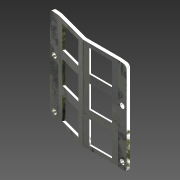
# Autodesk Inventor part: keyplate2
Saved by Autodesk Inventor 2018 (Build 220112000, 112)
## iProperties
Created: 2018-05-25
Part Number: keyplate2
Material: アルミニウム 6061
Document SubType Name: Sheet Metal
Designer: NaMACHAN
Mass: 8.70431 g
Surface Area: 50.6323 cm^2
Volume: 3.22382 cm^3
Density: 2.7 g/cm^3
Flat Pattern Width: 5.7 cm
Flat Pattern Length: 5.44568 cm
Flat Pattern Area: 31.0404 cm^2
Sheet Metal Rule: Al2mm
Sheet Metal Width: 57.000 mm
Sheet Metal Length: 54.457 mm
Sheet Metal Area: 3104.035 mm^2
Appearance: アルミニウム - フラット
Author: NaMACHAN
Autodesk Inventor part; units mm, degrees
ref_plane "YZ Plane" through (0, 0, 0) normal (1, 0, 0) x (0, 1, 0)
ref_plane "XZ Plane" through (0, 0, 0) normal (0, 1, 0) x (-1, 0, 0)
ref_plane "XY Plane" through (0, 0, 0) normal (0, 0, 1) x (1, 0, 0)
sketch "スケッチ1" plane through (0, 0, 0) normal (0, 1, 0) x (-1, 0, 0)
  line L0 (-10.5, -28.5) -> (10.5, -28.5)
  line L1 (10.5, -28.5) -> (10.5, 28.5)
  line L2 (10.5, 28.5) -> (-10.5, 28.5)
  line L3 (-10.5, 28.5) -> (-10.5, -28.5)
  line L4 (-10.5, -28.5) -> (10.5, 28.5) construction
  line L5 (10.5, -28.5) -> (-10.5, 28.5) construction
  line L6 (-7, 12) -> (7, 12)
  line L7 (7, 12) -> (7, 26)
  line L8 (7, 26) -> (-7, 26)
  line L9 (-7, 26) -> (-7, 12)
  line L10 (-7, 12) -> (7, 26) construction
  line L11 (7, 12) -> (-7, 26) construction
  line L12 (-7, -7) -> (7, -7)
  line L13 (7, -7) -> (7, 7)
  line L14 (7, 7) -> (-7, 7)
  line L15 (-7, 7) -> (-7, -7)
  line L16 (-7, -7) -> (7, 7) construction
  line L17 (7, -7) -> (-7, 7) construction
  line L18 (7, -26) -> (-7, -26)
  line L19 (-7, -26) -> (-7, -12)
  line L20 (-7, -12) -> (7, -12)
  line L21 (7, -12) -> (7, -26)
  line L22 (7, -26) -> (-7, -12) construction
  line L23 (-7, -26) -> (7, -12) construction
  point P0 (0, 0)
  point P1 (0, 19)
  point P2 (0, 0)
  point P3 (0, 0)
  point P4 (0, 0)
  point P5 (0, 19)
  point P6 (0, -19)
  point P7 (0, -19)
  dimension "d0" = 21
  dimension "d1" = 57
  dimension "d2" = 14
  dimension "d3" = 14
  dimension "d345" = 14
  dimension "d346" = 14
  dimension "d391" = 19
  dimension "d393" = 19
  dimension "d410" = 14
  dimension "d411" = 14
  dimension "d412" = 19
  measures "d0" distance of L2.end L1.end
  measures "d1" distance of L1.end L0.end
  measures "d2" distance of L8.end L7.end
  measures "d3" distance of L7.end L6.end
  measures "d345" distance of L14.end L13.end
  measures "d346" distance of L13.end L12.end
  measures "d391" distance of point (0, 19) point (0, 0)
  measures "d393" distance of point (0, 19) point (0, 0)
  measures "d410" distance of L19.end L20.end
  measures "d411" distance of L18.end L19.end
  measures "d412" distance of point (0, 0) point (0, -19)
extrude "プレート1" add sketch "スケッチ1" along normal blind 2
sketch "スケッチ2" plane through (-11.0176, 2.0681, 28.5) normal (-0.258819, -0.9659258, 0) x (0.9659258, -0.258819, 0)
  line L0 (0, -57) -> (0, 0)
  line L1 (0, 0) -> (-20.4734, 0)
  line L2 (-20.4734, 0) -> (-20.4734, -57)
  line L3 (-20.4734, -57) -> (0, -57)
  constraints: 6 end point, 1 horizontal, 1 perpendicular, 1 vertical
edge flange "フランジ1" height 21 angle 15 thickness 2 bend radius 2 thickness toward (-0.258819, -0.9659258, 0) relief tear relief width 2 relief depth 1 edges at (-10.5, 2, 0) wall of the first edge with corners at (-11.0176, 2.0681, -28.5) (-11.0176, 2.0681, 28.5) (-30.7934, 7.3671, 28.5) (-30.7934, 7.3671, -28.5)
bend "曲げ1"
corner "コーナー1"
sketch "スケッチ9" plane through (-11.0176, 2.0681, 28.5) normal (0.258819, 0.9659258, 0) x (0.9659258, -0.258819, 0)
  line L0 (-20.4734, 0) -> (0, 0) projected
  line L1 (-20.4734, 57) -> (-20.4734, 0) projected
  line L2 (0, 0) -> (0, 57) projected
  line L3 (-3.2367, 2.5) -> (-17.2367, 2.5)
  line L4 (-17.2367, 2.5) -> (-17.2367, 16.5)
  line L5 (-17.2367, 16.5) -> (-3.2367, 16.5)
  line L6 (-3.2367, 16.5) -> (-3.2367, 2.5)
  line L7 (-3.2367, 2.5) -> (-17.2367, 16.5) construction
  line L8 (-17.2367, 2.5) -> (-3.2367, 16.5) construction
  line L9 (-3.2367, 40.5) -> (-17.2367, 40.5)
  line L10 (-17.2367, 40.5) -> (-17.2367, 54.5)
  line L11 (-17.2367, 54.5) -> (-3.2367, 54.5)
  line L12 (-3.2367, 54.5) -> (-3.2367, 40.5)
  line L13 (-3.2367, 40.5) -> (-17.2367, 54.5) construction
  line L14 (-17.2367, 40.5) -> (-3.2367, 54.5) construction
  line L15 (-20.4734, 57) -> (0, 57) projected
  line L16 (-17.2367, 35.5) -> (-3.2367, 35.5)
  line L17 (-3.2367, 35.5) -> (-3.2367, 21.5)
  line L18 (-3.2367, 21.5) -> (-17.2367, 21.5)
  line L19 (-17.2367, 21.5) -> (-17.2367, 35.5)
  line L20 (-17.2367, 35.5) -> (-3.2367, 21.5) construction
  line L21 (-3.2367, 35.5) -> (-17.2367, 21.5) construction
  point P0 (11.1775, 28.5)
  point P1 (-10.2367, 0)
  point P2 (-10.2367, 9.5)
  point P3 (-10.2367, 47.5)
  point P4 (-10.2367, 47.5)
  point P5 (-10.2367, 9.5)
  point P6 (-3.2367, 9.5)
  point P7 (-10.2367, 9.5)
  point P8 (-10.2367, 0)
  point P9 (-10.2367, 28.5)
  point P10 (-10.2367, 28.5)
  dimension "d352" = 14
  dimension "d353" = 14
  dimension "d394" = 9.5
  dimension "d395" = 9.5
  dimension "d396" = 14
  dimension "d416" = 14
  dimension "d417" = 14
  dimension "d418" = 19
  constraints: 36 end point, 13 midpoint, 6 parallel, 3 horizontal, 3 perpendicular, 3 vertical alignment, 1 point on line
  measures "d352" distance of L9.end L10.end
  measures "d353" distance of L3.end L4.end
  measures "d394" distance from line of point (-10.237, 9.5) L0
  measures "d395" distance from line of L15 point (-10.237, 47.5)
  measures "d396" distance of L3.start L3.end
  measures "d416" distance of L17.end L18.end
  measures "d417" distance of L16.end L17.end
  measures "d418" distance of point (-10.237, 9.5) point (-10.237, 28.5)
extrude "押し出し3" cut sketch "スケッチ9" against normal blind 10 contours L3 L4 L5 L6 | L9 L10 L11 L12 | L16 L17 L18 L19
sketch "スケッチ26" plane through (-31.6544, 5.4957, -28.5) normal (0.0871557, 0.9961947, 0) x (-0.9961947, 0.0871557, 0)
  line L0 (0, 57) -> (0, 0)
  line L1 (0, 0) -> (5.65, 0)
  line L2 (5.65, 0) -> (5.65, 57)
  line L3 (5.65, 57) -> (0, 57)
  constraints: 6 end point, 1 horizontal, 1 perpendicular, 1 vertical
edge flange "フランジ13" height 6 angle 10 thickness 2 bend radius 2 thickness toward (0.0871557, 0.9961947, 0) relief tear relief width 2 relief depth 1 edges at (-31.3111, 5.4352, 0) wall of the first edge with corners at (-31.6544, 5.4957, 28.5) (-31.6544, 5.4957, -28.5) (-37.2829, 5.9882, -28.5) (-37.2829, 5.9882, 28.5)
bend "曲げ13"
corner "コーナー13"
sketch "スケッチ33" plane through (0, 2, 0) normal (0, 1, 0) x (1, 0, 0)
  line L0 (8, -11) -> (-8, -11)
  line L1 (-8, -11) -> (-8, -27)
  line L2 (-8, -27) -> (8, -27)
  line L3 (8, -27) -> (8, -11)
  line L4 (8, -11) -> (-8, -27) construction
  line L5 (-8, -11) -> (8, -27) construction
  line L6 (8, -8) -> (-8, -8)
  line L7 (-8, -8) -> (-8, 8)
  line L8 (-8, 8) -> (8, 8)
  line L9 (8, 8) -> (8, -8)
  line L10 (8, -8) -> (-8, 8) construction
  line L11 (-8, -8) -> (8, 8) construction
  line L12 (7, 7) -> (7, -7) projected
  line L13 (-7, -26) -> (-7, -12) projected
  line L14 (-7, -7) -> (-7, 7) projected
  line L15 (7, -26) -> (-7, -26) projected
  line L16 (-8, 27) -> (8, 27)
  line L17 (8, 27) -> (8, 11)
  line L18 (8, 11) -> (-8, 11)
  line L19 (-8, 11) -> (-8, 27)
  line L20 (-8, 27) -> (8, 11) construction
  line L21 (8, 27) -> (-8, 11) construction
  point P0 (0, -19)
  point P1 (0, 0)
  point P2 (0, -19)
  point P3 (0, -19)
  point P4 (0, 0)
  point P5 (0, 0)
  point P6 (7, 0)
  point P7 (-7, -19)
  point P8 (-7, 0)
  point P9 (0, -26)
  point P10 (0, 19)
  point P11 (0, 19)
  dimension "d265" = 16
  dimension "d266" = 16
  dimension "d356" = 16
  dimension "d357" = 16
  dimension "d413" = 16
  dimension "d414" = 16
  dimension "d415" = 19
  constraints: 36 end point, 15 midpoint, 6 parallel, 3 horizontal, 3 horizontal alignment, 3 perpendicular, 3 vertical alignment
  measures "d265" distance of L2.end L1.end
  measures "d266" distance of L1.end L0.end
  measures "d356" distance of L7.end L8.end
  measures "d357" distance of L6.end L7.end
  measures "d413" distance of L17.end L18.end
  measures "d414" distance of L16.end L17.end
  measures "d415" distance of point (0, 19) point (0, 0)
extrude "押し出し11" cut sketch "スケッチ33" against normal blind 1.6
sketch "スケッチ34" plane through (-11.0176, 2.0681, 28.5) normal (0.258819, 0.9659258, 0) x (0.9659258, -0.258819, 0)
  line L0 (-18.2367, 17.5) -> (-2.2367, 17.5)
  line L1 (-2.2367, 17.5) -> (-2.2367, 1.5)
  line L2 (-2.2367, 1.5) -> (-18.2367, 1.5)
  line L3 (-18.2367, 1.5) -> (-18.2367, 17.5)
  line L4 (-18.2367, 17.5) -> (-2.2367, 1.5) construction
  line L5 (-2.2367, 17.5) -> (-18.2367, 1.5) construction
  line L6 (-18.2367, 55.5) -> (-2.2367, 55.5)
  line L7 (-2.2367, 55.5) -> (-2.2367, 39.5)
  line L8 (-2.2367, 39.5) -> (-18.2367, 39.5)
  line L9 (-18.2367, 39.5) -> (-18.2367, 55.5)
  line L10 (-18.2367, 55.5) -> (-2.2367, 39.5) construction
  line L11 (-2.2367, 55.5) -> (-18.2367, 39.5) construction
  line L12 (-3.2367, 2.5) -> (-17.2367, 2.5) projected
  line L13 (-3.2367, 40.5) -> (-17.2367, 40.5) projected
  line L14 (-17.2367, 2.5) -> (-17.2367, 16.5) projected
  line L15 (-17.2367, 40.5) -> (-17.2367, 54.5) projected
  line L16 (-18.2367, 36.5) -> (-2.2367, 36.5)
  line L17 (-2.2367, 36.5) -> (-2.2367, 20.5)
  line L18 (-2.2367, 20.5) -> (-18.2367, 20.5)
  line L19 (-18.2367, 20.5) -> (-18.2367, 36.5)
  line L20 (-18.2367, 36.5) -> (-2.2367, 20.5) construction
  line L21 (-2.2367, 36.5) -> (-18.2367, 20.5) construction
  line L22 (-17.2367, 21.5) -> (-17.2367, 35.5) projected
  line L23 (-3.2367, 21.5) -> (-17.2367, 21.5) projected
  point P0 (11.1775, 28.5)
  point P1 (-3.5, 0)
  point P2 (-10.2367, 9.5)
  point P3 (-10.2367, 47.5)
  point P4 (-10.2367, 9.5)
  point P5 (-10.2367, 2.5)
  point P6 (-10.2367, 47.5)
  point P7 (-10.2367, 40.5)
  point P8 (-10.2367, 9.5)
  point P9 (-17.2367, 9.5)
  point P10 (-10.2367, 47.5)
  point P11 (-17.2367, 47.5)
  point P12 (-10.2367, 28.5)
  point P13 (-10.2367, 28.5)
  point P14 (-17.2367, 28.5)
  point P15 (-10.2367, 28.5)
  point P16 (-10.2367, 21.5)
  dimension "d397" = 16
  dimension "d398" = 16
  dimension "d399" = 16
  dimension "d419" = 16
  dimension "d420" = 16
  constraints: 36 end point, 18 midpoint, 6 parallel, 4 vertical alignment, 3 horizontal, 3 horizontal alignment, 3 perpendicular
  measures "d397" distance of L1.end L2.end
  measures "d398" distance of L2.end L0.start
  measures "d399" distance of L8.end L6.start
  measures "d419" distance of L17.end L18.end
  measures "d420" distance of L16.end L17.end
extrude "押し出し12" cut sketch "スケッチ34" against normal blind 1.6
sketch "スケッチ41" plane through (10.6743, -0.0076, 28.5) normal (0.0871557, 0.9961947, 0) x (-0.9961947, 0.0871557, 0)
  line L0 (0, -57) -> (0, 0)
  line L1 (0, 0) -> (-5.8254, 0)
  line L2 (-5.8254, 0) -> (-5.8254, -57)
  line L3 (-5.8254, -57) -> (0, -57)
  constraints: 6 end point, 1 horizontal, 1 perpendicular, 1 vertical
edge flange "フランジ18" height 6 angle 5 thickness 2 bend radius 2 thickness toward (0.0871557, 0.9961947, 0) relief tear relief width 2 relief depth 1 edges at (10.5, 0, 0) wall of the first edge with corners at (10.6743, -0.0076, -28.5) (10.6743, -0.0076, 28.5) (16.4775, -0.5153, 28.5) (16.4775, -0.5153, -28.5)
bend "曲げ19"
corner "コーナー18"
sketch "スケッチ43" plane through (10.8486, 1.9848, 28.5) normal (0.0871557, 0.9961947, 0) x (0, 0, -1)
  line L0 (0, -5.8254) -> (0, 0) projected
  line L1 (57, 0) -> (57, -5.8254) projected
  point P0 (28.5, 10.6344)
  point P1 (23, -2.9127)
  point P2 (0, -2.9127)
  point P3 (53, -2.9127)
  point P4 (57, -2.9127)
  dimension "d441" = 30
  dimension "d445" = 4
  constraints: 2 horizontal alignment, 2 midpoint
  measures "d441" distance of point (53, -2.913) point (23, -2.913)
  measures "d445" distance of point (57, -2.913) point (53, -2.913)
hole "穴8" at (13.7502, 1.7309, 5.5) at (13.7502, 1.7309, -24.5) direction (-0.0871557, -0.9961947, 0) diameter 3 end through all
fillet "コーナーR5" radius 2 4 edges at (16.5647, 0.4809, -28.5) (16.5647, 0.4809, 28.5) (-37.1958, 6.9844, 28.5) (-37.1958, 6.9844, -28.5)
sketch "スケッチ48" plane through (-31.4801, 7.4881, 28.5) normal (0.0871557, 0.9961947, 0) x (0.9961947, -0.0871557, 0)
  line L0 (0, 0) -> (-3.65, 0) projected
  line L1 (-5.65, 2) -> (-5.65, 55) projected
  line L2 (-3.65, 57) -> (0, 57) projected
  point P0 (32.0129, 28.5)
  point P1 (-2.65, 23)
  point P2 (-2.65, 53)
  dimension "d437" = 3
  dimension "d443" = 30
  dimension "d444" = 3
  dimension "d446" = 4
  measures "d437" distance from line of L1 point (-2.65, 23)
  measures "d443" distance of point (-2.65, 53) point (-2.65, 23)
  measures "d444" distance from line of L1 point (-2.65, 53)
  measures "d446" distance from line of L2 point (-2.65, 53)
hole "穴9" at (-34.12, 7.7191, 5.5) at (-34.12, 7.7191, -24.5) direction (-0.0871557, -0.9961947, 0) diameter 3 end through all
equation "\"d4\" = Thickness"
equation "\"d5\" = BendReliefWidth"
equation "\"d6\" = BendReliefDepth"
equation "\"d7\" = MinimumRemnant"
equation "\"d8\" = TransitionRadius"
equation "\"d11\" = BendRadius"
equation "\"d12\" = CornerReliefSize"
equation "\"d13\" = GapSize"
equation "\"d14\" = JacobiRadiusSize"
equation "\"d205\" = BendReliefWidth"
equation "\"d206\" = BendReliefDepth"
equation "\"d207\" = MinimumRemnant"
equation "\"d208\" = TransitionRadius"
equation "\"d211\" = BendRadius"
equation "\"d212\" = CornerReliefSize"
equation "\"d213\" = GapSize"
equation "\"d214\" = JacobiRadiusSize"
equation "\"BendRadius\" = Thickness"
equation "\"BendReliefWidth\" = Thickness"
equation "\"BendReliefDepth\" = 0.5 * Thickness"
equation "\"CornerReliefSize\" = 4 * Thickness"
equation "\"MinimumRemnant\" = 2 * Thickness"
equation "\"TransitionRadius\" = BendRadius"
equation "\"JacobiRadiusSize\" = BendRadius"
equation "\"GapSize\" = Thickness"
equation "\"Thickness\" = 2"
